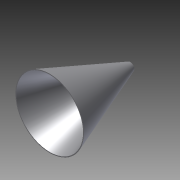
# Autodesk Inventor part: Tube
Saved by Autodesk Inventor 2012 (Build 160160000, 160)
## iProperties
Created: 2011-08-19
Part Number: Tube
Material: Default
Document SubType Name: Modeling
Designer: Minh Tran
Density: 1 g/cm^3
Author: Minh Tran
Autodesk Inventor part; units mm, degrees
ref_plane "YZ Plane" through (0, 0, 0) normal (1, 0, 0) x (0, 1, 0)
sketch "Sketch1" plane through (0, 0, 0) normal (0, 0, 1) x (1, 0, 0)
  circle A0 centre (0, 0) radius 12.7
  dimension "d0" = 25.4
  constraints: 1 centre point, 1 coincident
  measures "d0" diameter of A0
ref_plane "Work Plane1" through (0, 0, 254) normal (0, 0, 1) x (1, 0, 0)
ref_plane "Work Plane2" through (0, 0, 254) normal (0, 0, 1) x (1, 0, 0)
sketch "Sketch3" plane through (0, 0, 254) normal (0, 0, 1) x (1, 0, 0)
  circle A0 centre (0, 0) radius 107.95
  dimension "d9" = 215.9
  constraints: 1 centre point, 1 coincident
  measures "d9" diameter of A0
loft "Loft2" add profiles "Sketch3", "Sketch1"
shell "Shell2" thickness 2.54 removed faces 2 at (-32.0495, 20.0441, 254) at (-3.6254, -0.9542, 0)
body "Solid2"
